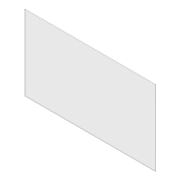
# Autodesk Inventor part: FE-00012
Saved by Autodesk Inventor 2012 (Build 160160000, 160)
## iProperties
Created: 2008-06-02
Part Number: FE-00012
Document SubType Name: Modeling
Designer: mcyr
Density: 1 g/cm^3
Description: Drivers Station Acrylic
Mass: 18361.7 g
Surface Area: 39104 cm^2
Volume: 18361.7 cm^3
Material: Default
Title: FE-00012
Author: mcyr
Autodesk Inventor part; units mm, degrees
ref_plane "YZ Plane" through (0, 0, 0) normal (1, 0, 0) x (0, 1, 0)
ref_plane "XZ Plane" through (0, 0, 0) normal (0, 1, 0) x (-1, 0, 0)
ref_plane "XY Plane" through (0, 0, 0) normal (0, 0, 1) x (1, 0, 0)
sketch "Sketch1" plane through (0, 0, 0) normal (0, 0, 1) x (1, 0, 0)
  line L0 (-44.4023, 0) -> (1784.3977, 0)
  line L1 (1784.3977, 0) -> (1784.3977, 1054.1)
  line L2 (1784.3977, 1054.1) -> (-44.4023, 1054.1)
  line L3 (-44.4023, 1054.1) -> (-44.4023, 0)
  dimension "d0" = 1828.8
  dimension "d1" = 1054.1
  constraints: 8 end point, 2 parallel, 1 horizontal, 1 perpendicular
  measures "d0" distance of L0.start L0.end
  measures "d1" distance of L2.end L0.start
extrude "Extrusion1" add sketch "Sketch1" along normal blind 9.525
body "Solid1"
